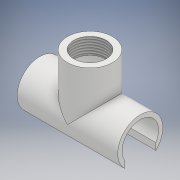
# Autodesk Inventor part: Piping_TeeInline_1in
Saved by Autodesk Inventor 2018 (Build 220112000, 112)
## iProperties
Created: 2018-10-12
Part Number: Piping_TeeInline_1in
Material: PVC-Piping
Document SubType Name: Modeling
Designer: Bradley
Density: 1.4 g/cm^3
Appearance: Smooth - White
Author: Bradley
Autodesk Inventor part; units mm, degrees
ref_plane "YZ Plane" through (0, 0, 0) normal (1, 0, 0) x (0, 1, 0)
ref_plane "XZ Plane" through (0, 0, 0) normal (0, 1, 0) x (-1, 0, 0)
sketch "Sketch1" plane through (0, 0, 0) normal (1, 0, 0) x (0, 1, 0)
  circle A0 centre (0, 0) radius 20.6375
  circle A1 centre (0, 0) radius 16.7005
  line L0 (-14.2875, -8.6472) -> (-14.2875, -14.8921)
  line L1 (14.2875, -8.6472) -> (14.2875, -14.8921)
  dimension "d0" = 41.275
  dimension "d1" = 33.401
  dimension "d2" = 28.575
  constraints: 4 end point, 4 point on circle, 2 centre point, 2 coincident, 2 parallel, 1 vertical
  measures "d0" diameter of A0
  measures "d1" diameter of A1
  measures "d2" distance between parallel lines of L1 L0
extrude "Extrusion1" add sketch "Sketch1" along normal mid plane 92.075 contours A0 L1 A1 L0 picked at (-15.3557, -11.497)
ref_plane "Work Plane1" through (0, 0, 49.2125) normal (0, 0, 1) x (1, 0, 0)
sketch "Sketch2" plane through (0, 0, 49.2125) normal (0, 0, 1) x (1, 0, 0)
  line L0 (-46.0375, 20.6375) -> (46.0375, 20.6375) projected
  circle A0 centre (0, 0) radius 20.6375
  constraints: 1 centre point, 1 coincident, 1 tangent
extrude "Extrusion2" add sketch "Sketch2" against normal up to next
hole "Hole1" at (0, 0, 49.2125) direction (0, 0, -1) diameter 28.575 end through all taper from width 29.6938 to width 28.783 over 14.577 thread size "1" designation "1 - 11.5 NPT" standard "NPT for PVC Pipe and Fitting"
body "Solid1"
